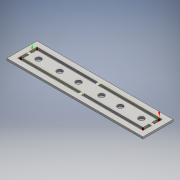
# Autodesk Inventor part: side
Saved by Autodesk Inventor 2016 (Build 200138000, 138)
## iProperties
Created: 2016-09-24
Part Number: side
Material: Generic
Document SubType Name: Modeling
Designer: Kevin G
Density: 1 g/cm^3
Appearance: Default
Author: Kevin G
Autodesk Inventor part; units mm, degrees
ref_plane "YZ Plane" through (0, 0, 0) normal (1, 0, 0) x (0, 1, 0)
ref_plane "XZ Plane" through (0, 0, 0) normal (0, 1, 0) x (-1, 0, 0)
ref_plane "XY Plane" through (0, 0, 0) normal (0, 0, 1) x (1, 0, 0)
sketch "Sketch1" plane through (0, 0, 0) normal (0, 0, 1) x (1, 0, 0)
  line L0 (469.9, 22.205) -> (469.9, -34.945)
  line L1 (-99.06, -34.945) -> (-99.06, 22.205)
  circle A0 centre (-58.42, -4.7925) radius 13
  circle A1 centre (41.716, -4.7925) radius 13
  circle A2 centre (131.092, -4.7925) radius 13
  circle A3 centre (429.26, -4.7925) radius 13
  circle A4 centre (329.124, -4.7925) radius 13
  circle A5 centre (239.748, -4.7925) radius 13
  line L2 (-99.06, 28.36) -> (469.9, 28.36)
  line L3 (-99.06, -37.945) -> (469.9, -37.945)
  line L4 (-99.06, 22.205) -> (-99.06, 28.36)
  line L5 (-99.06, -37.945) -> (-99.06, -34.945)
  line L6 (469.9, -37.945) -> (469.9, -34.945)
  line L7 (469.9, 22.205) -> (469.9, 28.36)
  line L8 (-111.76, 41.06) -> (482.6, 41.06)
  line L9 (482.6, 41.06) -> (482.6, -50.645)
  line L10 (482.6, -50.645) -> (-111.76, -50.645)
  line L11 (-111.76, -50.645) -> (-111.76, 41.06)
  line L12 (508, 63.305) -> (508, -76.045)
  line L13 (508, -76.045) -> (-137.16, -76.045)
  line L14 (-137.16, -76.045) -> (-137.16, 63.305)
  line L15 (170, 41.06) -> (170, 66.46)
  line L16 (-137.16, 66.46) -> (508, 66.46)
  line L17 (508, 66.46) -> (508, 63.305)
  line L18 (-137.16, 66.46) -> (-137.16, 62)
  line L19 (-99.06, 4) -> (-111.76, 4)
  line L20 (-99.06, -10) -> (-111.76, -10)
  line L21 (176, 28.36) -> (176, 41.06)
  line L22 (191, 28.36) -> (191, 41.06)
  line L23 (176, -37.945) -> (176, -50.645)
  line L24 (191, -37.945) -> (191, -50.645)
  line L25 (469.9, 4) -> (482.6, 4)
  line L26 (469.9, -10) -> (482.6, -10)
  point P0 (0, 0)
  dimension "d4" = 26
  dimension "d6" = 26
  dimension "d8" = 26
  dimension "d10" = 26
  dimension "d12" = 26
  dimension "d14" = 26
  dimension "d16" = 568.96
  dimension "d18" = 40.64
  dimension "d19" = 140.776
  dimension "d20" = 230.152
  dimension "d21" = 230.152
  dimension "d22" = 40.64
  dimension "d23" = 140.776
  dimension "d29" = 66.305
  dimension "d45" = 33.1525
  dimension "d46" = 33.1525
  dimension "d47" = 33.1525
  dimension "d48" = 33.1525
  dimension "d49" = 33.1525
  dimension "d50" = 33.1525
  dimension "d52" = 12.7
  dimension "d53" = 12.7
  dimension "d54" = 25.4
  dimension "d56" = 25.4
  dimension "d57" = 15
  constraints: 54 end point, 22 point on line, 7 parallel, 7 perpendicular, 6 centre point, 4 horizontal, 1 collinear, 1 vertical
  measures "d4" diameter of A0
  measures "d6" diameter of A1
  measures "d8" diameter of A2
  measures "d10" diameter of A3
  measures "d12" diameter of A4
  measures "d14" diameter of A5
  measures "d16" distance between parallel lines of L0 L1
  measures "d18" distance from line of A0.centre L1
  measures "d19" distance from line of A1.centre L1
  measures "d20" distance from line of A2.centre L1
  measures "d21" distance from line of A5.centre L0
  measures "d22" distance from line of A3.centre L0
  measures "d23" distance from line of A4.centre L0
  measures "d29" distance between parallel lines of L2 L3
  measures "d45" distance from line of L3 A0.centre
  measures "d46" distance from line of L3 A1.centre
  measures "d47" distance from line of L3 A2.centre
  measures "d48" distance from line of L3 A5.centre
  measures "d49" distance from line of L3 A4.centre
  measures "d50" distance from line of L3 A3.centre
  measures "d52" distance between parallel lines of L8 L2
  measures "d53" distance between parallel lines of L10 L3
  measures "d54" distance between parallel lines of L13 L10
  measures "d56" distance of L15.end L15.start
  measures "d57" distance between parallel lines of L22 L21
extrude "Extrusion4" add sketch "Sketch1" along normal blind 9.525 contours L0 L6 L3 L5 L1 L4 L2 L7 | L25 L9 L26 L0 | L16 L17 L12 L13 L14 L18 | L2 L21 L8 L22 | L24 L10 L23 L3 | L1 L20 L11 L19
body "Solid4"
